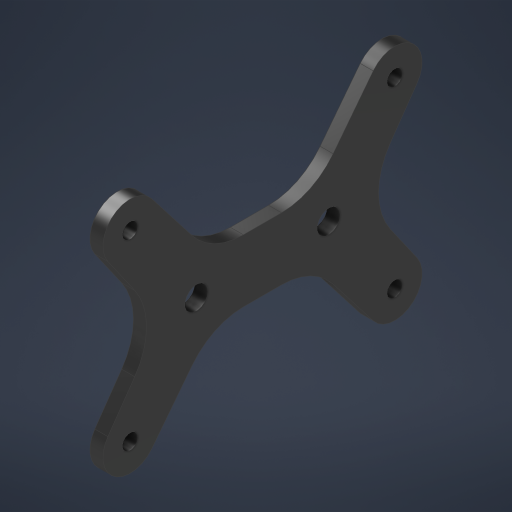
# Autodesk Inventor part: pump mount
Saved by Autodesk Inventor 2024 (Build 280153000, 153)
## iProperties
Created: 2025-02-16
Part Number: pump mount
Material: Generic
Document SubType Name: Modeling
Designer: Vincent Larson
Density: 1 g/cm^3
Appearance: Default
Author: Vincent Larson
## iProperties of the stored document pump mount_3DPrint.ipt
Created: 2025-02-24
Part Number: pump mount_3DPrint
Material: Generic
Document SubType Name: Modeling
Designer: Vincent Larson
Density: 1 g/cm^3
Appearance: Default
Author: Vincent Larson
Autodesk Inventor part; units mm, degrees
ref_plane "YZ Plane" through (0, 0, 0) normal (1, 0, 0) x (0, 1, 0)
ref_plane "XZ Plane" through (0, 0, 0) normal (0, 1, 0) x (-1, 0, 0)
ref_plane "XY Plane" through (0, 0, 0) normal (0, 0, 1) x (1, 0, 0)
sketch "Sketch1" plane through (0, 0, 0) normal (1, 0, 0) x (0, 1, 0)
  circle A0 centre (0, 0) radius 1.5
  line L0 (0, 0) -> (-35.6, 0)
  circle A1 centre (-35.6, 0) radius 1.5
  line L1 (0, 0) -> (0, -51.5)
  circle A2 centre (0, -51.5) radius 1.5
  circle A3 centre (-35.6, -51.5) radius 1.5
  line L2 (0, 0) -> (-35.6, 0)
  line L3 (-35.6, 0) -> (-35.6, -51.5)
  line L4 (-35.6, -51.5) -> (0, -51.5)
  line L5 (0, -51.5) -> (0, 0)
  line L6 (-17.8, 0) -> (-17.8, -51.5)
  line L7 (-17.8, -25.75) -> (-17.8, 0)
  line L8 (-17.8, -12.875) -> (-17.8, -51.5)
  line L9 (-17.8, -25.75) -> (-17.8, -51.5)
  line L10 (-17.8, -38.625) -> (-17.8, -12.875)
  circle A4 centre (-17.8, -12.875) radius 2.25
  circle A5 centre (-17.8, -38.625) radius 2.25
  line L11 (-15.9797, -9.3512) -> (-0.86, 1.229)
  line L12 (-19.6203, -9.3512) -> (-34.74, 1.229)
  line L13 (-15.55, -15.4984) -> (-15.55, -36.0016)
  line L14 (-20.05, -36.0016) -> (-20.05, -15.4984)
  line L15 (-19.6203, -42.1488) -> (-34.74, -52.729)
  line L16 (-21.2808, -38.5117) -> (-36.5185, -50.3141)
  line L17 (-21.2808, -12.9883) -> (-36.5185, -1.1859)
  line L18 (-14.3192, -12.9883) -> (0.9185, -1.1859)
  line L19 (-14.3192, -38.5117) -> (0.9185, -50.3141)
  line L20 (-15.9797, -42.1488) -> (-0.86, -52.729)
  arc A6 (-14.3192, -12.9883) -> (-15.55, -15.4984) centre (-12.375, -15.4984) ccw
  arc A7 (-15.55, -36.0016) -> (-14.3192, -38.5117) centre (-12.375, -36.0016) ccw
  arc A8 (-21.2808, -38.5117) -> (-20.05, -36.0016) centre (-23.225, -36.0016) ccw
  arc A9 (-20.05, -15.4984) -> (-21.2808, -12.9883) centre (-23.225, -15.4984) ccw
  arc A10 (-19.6203, -9.3512) -> (-15.9797, -9.3512) centre (-17.8, -6.7499) ccw
  arc A11 (-15.9797, -42.1488) -> (-19.6203, -42.1488) centre (-17.8, -44.7501) ccw
  line L21 (1.6962, -2.1899) -> (-13.5415, -13.9923)
  arc A12 (-13.5415, -13.9923) -> (-14.28, -15.4984) centre (-12.375, -15.4984) ccw
  line L22 (-14.28, -15.4984) -> (-14.28, -36.0016)
  arc A13 (-14.28, -36.0016) -> (-13.5415, -37.5077) centre (-12.375, -36.0016) ccw
  line L23 (-13.5415, -37.5077) -> (1.6962, -49.3101)
  line L24 (-37.2962, -2.1899) -> (-22.0585, -13.9923)
  arc A14 (-21.32, -15.4984) -> (-22.0585, -13.9923) centre (-23.225, -15.4984) ccw
  line L25 (-21.32, -15.4984) -> (-21.32, -36.0016)
  arc A15 (-22.0585, -37.5077) -> (-21.32, -36.0016) centre (-23.225, -36.0016) ccw
  line L26 (-22.0585, -37.5077) -> (-37.2962, -49.3101)
  line L27 (-1.5881, 2.2695) -> (-16.7078, -8.3107)
  arc A16 (-18.8922, -8.3107) -> (-16.7078, -8.3107) centre (-17.8, -6.7499) ccw
  line L28 (-18.8922, -8.3107) -> (-34.0119, 2.2695)
  circle A17 centre (0, 0) radius 2.77
  circle A18 centre (-17.8, -12.875) radius 3.52
  circle A19 centre (-17.8, -38.625) radius 3.52
  circle A20 centre (-35.6, 0) radius 2.77
  circle A21 centre (-35.6, -51.5) radius 2.77
  circle A22 centre (0, -51.5) radius 2.77
  line L29 (-1.5881, -53.7695) -> (-16.7078, -43.1893)
  arc A23 (-16.7078, -43.1893) -> (-18.8922, -43.1893) centre (-17.8, -44.7501) ccw
  line L30 (-18.8922, -43.1893) -> (-34.0119, -53.7695)
  point P0 (-17.8, -10.625)
  point P1 (-15.55, -12.875)
  point P2 (-15.55, -38.625)
  point P3 (-20.05, -38.625)
  point P4 (-20.05, -12.875)
  point P5 (-17.8, -40.875)
  point P6 (-18.8754, -36.6486)
  point P7 (-18.8754, -14.8514)
  point P8 (-16.7246, -14.8514)
  point P9 (-16.7246, -36.6486)
  point P10 (-34.0119, 2.2695)
  point P11 (1.6962, -49.3101)
  dimension "d0" = 3
  dimension "d1" = 35.6
  dimension "d2" = 51.5
  dimension "d3" = 4.5
  dimension "d4" = 3.175
  dimension "d5" = 1.27
  dimension "d6" = 1.27
  dimension "d7" = 1.27
  dimension "d8" = 1.27
  dimension "d9" = 1.27
  dimension "d10" = 1.27
  dimension "d11" = 1.27
  dimension "d12" = 1.27
  dimension "d13" = 1.27
  dimension "d14" = 1.27
  constraints: 62 end point, 42 point on circle, 24 centre point, 23 tangent, 14 point on line, 5 coincident, 5 equal radius, 5 midpoint, 4 collinear, 2 horizontal, 2 parallel, 1 perpendicular, 1 vertical, 12 other
  measures "d0" diameter of A0
  measures "d1" distance of L0.start L0.end
  measures "d2" distance of L0.start L1.end
  measures "d3" diameter of A4
  measures "d4" radius of A6
  measures "d5" distance between parallel lines of L18 L21
  measures "d6" distance between parallel lines of L14 L25
  measures "d7" distance between parallel lines of L11 L27
  measures "d8" radial gap between concentric circles of A0 A17
  measures "d9" radial gap between concentric circles of A4 A18
  measures "d10" radial gap between concentric circles of A5 A19
  measures "d11" radial gap between concentric circles of A1 A20
  measures "d12" radial gap between concentric circles of A3 A21
  measures "d13" radial gap between concentric circles of A2 A22
  measures "d14" distance between parallel lines of L20 L29
extrude "Extrusion1" add sketch "Sketch1" along normal blind 2.54 contours A0 L11 L0 A17 L1 L18 | A0 L0 L11 | L18 L1 A0 | A0 L1 L18 A17 L11 L0 | L11 A17 L0 | L1 A17 L18 | A17 L11 A10 A18 L6 A16 L27 L0 | L0 L27 A17 | A17 L18 A18 A10 L11 | A17 L21 L1 | L1 L21 A12 L22 A13 L23 A22 L19 A19 L13 A18 L18 A17 | A18 L13 A6 L18 | L18 A6 L13 A18 L6 A4 A10 | A10 L6 A18 | L23 A22 L1 | L13 A19 L6 A18 | L28 A16 L6 A18 A10 L12 A20 L0 | L0 A20 L28 | A10 A18 L6 | L6 A4 A18 L14 A9 L17 A10 | A22 L4 L20 A2 L19 L1 | L1 L19 A22 | A19 L19 A7 L13 | L13 A7 L19 A19 A11 L6 A5 | L6 A19 L14 A18 | A20 L12 L0 | L0 L12 A1 L17 L3 A20 | A18 L17 A20 L12 A10 | L19 A2 L1 | L1 A2 L4 L20 A22 L19 | A22 L20 A11 A19 L19 | L6 A5 A11 A19 L16 A8 L14 | A18 L17 A9 L14 | L14 A19 L16 A21 L3 L26 A15 L25 A14 L24 A20 L17 A18 | L12 A20 L17 L3 A1 L0 | L0 A1 L12 | A20 L3 L24 | A22 L4 L29 A23 L6 A19 A11 L20 | L20 L4 A22 | L29 L4 A22 | L14 A8 L16 A19 | A20 L3 L17 | A2 L20 L4 | A19 L6 A11 | A19 A11 L15 A21 L16 | L3 L17 A1 | L3 A21 L26 | L6 A19 A11 | L6 A23 L30 L4 A21 L15 A11 A19 | A21 L15 L4 A3 L3 L16 | L16 L3 A21 | L3 L16 A3 L15 L4 A21 | L30 A21 L4 | L3 A3 L16 | A21 L4 L15 | L15 A3 L4
sketch "Sketch2" plane through (2.54, 0, 0) normal (1, 0, 0) x (0, 0, -1)
  circle A0 centre (0, 0) radius 1.5 projected
  circle A1 centre (0, 0) radius 1.5
  circle A2 centre (12.875, -17.8) radius 2.25 projected
  circle A3 centre (12.875, -17.8) radius 2.25
  circle A4 centre (38.625, -17.8) radius 2.25 projected
  circle A5 centre (38.625, -17.8) radius 2.25
  circle A6 centre (51.5, 0) radius 1.5 projected
  circle A7 centre (51.5, 0) radius 1.5
  circle A8 centre (51.5, -35.6) radius 1.5 projected
  circle A9 centre (51.5, -35.6) radius 1.5
  circle A10 centre (0, -35.6) radius 1.5 projected
  circle A11 centre (0, -35.6) radius 1.5
  line L0 (13.9923, -13.5415) -> (2.1899, 1.6962) projected
  arc A12 (2.1899, 1.6962) -> (-2.2695, -1.5881) centre (0, 0) ccw projected
  arc A13 (2.1899, 1.6962) -> (-2.2695, -1.5881) centre (0, 0) ccw
  arc A14 (53.7695, -1.5881) -> (49.3101, 1.6962) centre (51.5, 0) ccw projected
  arc A15 (53.7695, -1.5881) -> (49.3101, 1.6962) centre (51.5, 0) ccw
  arc A16 (49.3101, -37.2962) -> (53.7695, -34.0119) centre (51.5, -35.6) ccw projected
  arc A17 (49.3101, -37.2962) -> (53.7695, -34.0119) centre (51.5, -35.6) ccw
  arc A18 (-2.2695, -34.0119) -> (2.1899, -37.2962) centre (0, -35.6) ccw projected
  arc A19 (-2.2695, -34.0119) -> (2.1899, -37.2962) centre (0, -35.6) ccw
  arc A20 (15.4984, -21.32) -> (13.9923, -22.0585) centre (15.4984, -23.225) ccw projected
  arc A21 (15.4984, -21.32) -> (13.9923, -22.0585) centre (15.4984, -23.225) ccw
  arc A22 (8.3107, -18.8922) -> (8.3107, -16.7078) centre (6.7499, -17.8) ccw projected
  arc A23 (8.3107, -18.8922) -> (8.3107, -16.7078) centre (6.7499, -17.8) ccw
  arc A24 (13.9923, -13.5415) -> (15.4984, -14.28) centre (15.4984, -12.375) ccw projected
  arc A25 (13.9923, -13.5415) -> (15.4984, -14.28) centre (15.4984, -12.375) ccw
  arc A26 (36.0016, -14.28) -> (37.5077, -13.5415) centre (36.0016, -12.375) ccw projected
  arc A27 (36.0016, -14.28) -> (37.5077, -13.5415) centre (36.0016, -12.375) ccw
  arc A28 (37.5077, -22.0585) -> (36.0016, -21.32) centre (36.0016, -23.225) ccw projected
  arc A29 (37.5077, -22.0585) -> (36.0016, -21.32) centre (36.0016, -23.225) ccw
  arc A30 (43.1893, -16.7078) -> (43.1893, -18.8922) centre (44.7501, -17.8) ccw projected
  arc A31 (43.1893, -16.7078) -> (43.1893, -18.8922) centre (44.7501, -17.8) ccw
  line L1 (2.1899, 1.6962) -> (13.9923, -13.5415)
  line L2 (-2.2695, -1.5881) -> (8.3107, -16.7078) projected
  line L3 (8.3107, -16.7078) -> (-2.2695, -1.5881)
  line L4 (8.3107, -18.8922) -> (-2.2695, -34.0119) projected
  line L5 (8.3107, -18.8922) -> (-2.2695, -34.0119)
  line L6 (2.1899, -37.2962) -> (13.9923, -22.0585)
  line L7 (15.4984, -21.32) -> (36.0016, -21.32)
  line L8 (36.0016, -14.28) -> (15.4984, -14.28) projected
  line L9 (36.0016, -14.28) -> (15.4984, -14.28)
  line L10 (49.3101, 1.6962) -> (37.5077, -13.5415) projected
  line L11 (49.3101, 1.6962) -> (37.5077, -13.5415)
  line L12 (43.1893, -16.7078) -> (53.7695, -1.5881)
  line L13 (53.7695, -34.0119) -> (43.1893, -18.8922) projected
  line L14 (43.1893, -18.8922) -> (53.7695, -34.0119)
  line L15 (37.5077, -22.0585) -> (49.3101, -37.2962)
  arc A32 (-4.3506, -32.5556) -> (4.198, -38.8516) centre (0, -35.6) ccw
  line L16 (-4.3506, -32.5556) -> (5.9748, -17.8)
  line L17 (5.9748, -17.8) -> (-4.3506, -3.0444)
  arc A33 (4.198, 3.2516) -> (-4.3506, -3.0444) centre (0, 0) ccw
  line L18 (4.198, 3.2516) -> (15.8097, -11.74)
  line L19 (15.8097, -11.74) -> (35.6903, -11.74)
  line L20 (35.6903, -11.74) -> (47.302, 3.2516)
  arc A34 (55.8506, -3.0444) -> (47.302, 3.2516) centre (51.5, 0) ccw
  line L21 (47.302, -38.8516) -> (35.6903, -23.86)
  line L22 (35.6903, -23.86) -> (15.8097, -23.86)
  line L23 (15.8097, -23.86) -> (4.198, -38.8516)
  arc A35 (-4.3506, -32.5556) -> (4.198, -38.8516) centre (0, -35.6) ccw
  line L24 (35.4996, -11.9862) -> (47.302, 3.2516)
  arc A36 (55.8506, -3.0444) -> (47.302, 3.2516) centre (51.5, 0) ccw
  line L25 (55.8506, -3.0444) -> (45.5252, -17.8)
  line L26 (45.5252, -17.8) -> (55.8506, -32.5556)
  circle A37 centre (51.5, -35.6) radius 5.31
  point P0 (55.8506, -3.0444)
  point P1 (4.198, -38.8516)
  dimension "d17" = 2.54
  dimension "d18" = 2.54
  dimension "d19" = 2.54
  constraints: 42 end point, 36 point on circle, 21 centre point, 9 tangent, 7 coincident, 4 collinear, 2 concentric, 1 horizontal, 1 point on line, 16 other
  measures "d17" distance between parallel lines of L8 L19
  measures "d18" distance between parallel lines of L7 L22
  measures "d19" distance between parallel lines of L12 L25
extrude "Extrusion2" add sketch "Sketch2" against normal up to surface (2.54 mm away)
fillet "Fillet1" radius 12.7 6 edges at (1.27, -17.8, -5.9748) (1.27, -23.86, -15.8097) (1.27, -23.86, -35.6903) (1.27, -17.8, -45.5252) (1.27, -11.74, -35.6903) (1.27, -11.74, -15.8097)
body "Solid1"
